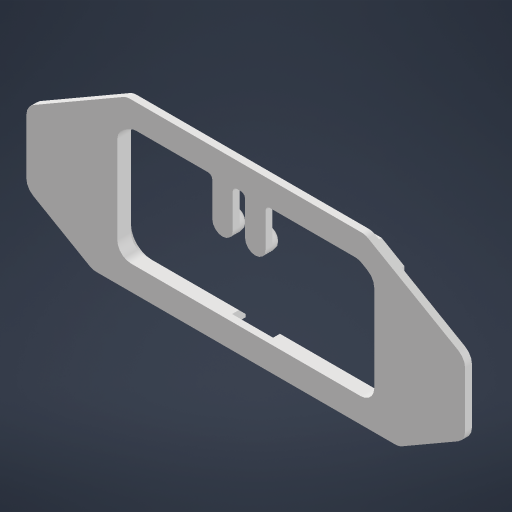
# Autodesk Inventor part: Joystick Top
Saved by Autodesk Inventor 2023.4 (Build 274418000, 418)
## iProperties
Created: 2024-04-17
Part Number: Joystick Top
Material: Generic
Document SubType Name: Modeling
Designer: xSibe
Density: 1 g/cm^3
Appearance: Default
Author: xSibe
Autodesk Inventor part; units mm, degrees
ref_plane "YZ Plane" through (0, 0, 0) normal (1, 0, 0) x (0, 1, 0)
ref_plane "XZ Plane" through (0, 0, 0) normal (0, 1, 0) x (-1, 0, 0)
ref_plane "XY Plane" through (0, 0, 0) normal (0, 0, 1) x (1, 0, 0)
ref_plane "Work Plane1" through (0, 0, 8.5) normal (0, 0, 1) x (1, 0, 0)
sketch "Sketch1" plane through (0, 0, 8.5) normal (0, 0, 1) x (1, 0, 0)
  line L0 (-3.75, -14) -> (-3.75, -11.5) projected
  line L1 (-25.5, -11.5) -> (-3.75, -11.5) projected
  line L2 (-25.5, 11.5) -> (-25.5, -11.5) projected
  line L3 (25.5, -11.5) -> (25.5, 11.5) projected
  line L4 (3.75, -11.5) -> (25.5, -11.5) projected
  line L5 (3.75, -11.5) -> (3.75, -14) projected
  line L6 (27.3301, -14) -> (3.75, -14) projected
  line L7 (-3.75, -14) -> (-27.3301, -14) projected
  line L8 (38.8744, -7.7217) -> (28.5801, -13.6651) projected
  line L9 (-28.5801, -13.6651) -> (-38.8744, -7.7217) projected
  line L10 (40.1244, 10.5622) -> (40.1244, -5.5566) projected
  line L11 (-40.1244, 10.5622) -> (-40.1244, -5.5566) projected
  line L12 (-21.1699, 14) -> (-25.5, 11.5) projected
  line L13 (21.1699, 14) -> (-21.1699, 14) projected
  line L14 (25.5, 11.5) -> (21.1699, 14) projected
  arc A0 (-28.5801, -13.6651) -> (-27.3301, -14) centre (-27.3301, -11.5) ccw projected
  arc A1 (27.3301, -14) -> (28.5801, -13.6651) centre (27.3301, -11.5) ccw projected
  arc A2 (38.8744, -7.7217) -> (40.1244, -5.5566) centre (37.6244, -5.5566) ccw projected
  arc A3 (-40.1244, -5.5566) -> (-38.8744, -7.7217) centre (-37.6244, -5.5566) ccw projected
  line L15 (25.5, -11.5) -> (-25.5, -11.5)
  line L16 (-25.5, -11.5) -> (-25.5, 11.5)
  line L17 (-25.5, 11.5) -> (-21.1699, 14)
  line L18 (-21.1699, 14) -> (21.1699, 14)
  line L19 (21.1699, 14) -> (25.5, 11.5)
  line L20 (25.5, 11.5) -> (25.5, -11.5)
  line L21 (-25.25, -11.25) -> (25.25, -11.25)
  line L22 (25.25, -11.25) -> (25.25, 11.3557)
  line L23 (25.25, 11.3557) -> (21.1029, 13.75)
  line L24 (21.1029, 13.75) -> (-21.1029, 13.75)
  line L25 (-21.1029, 13.75) -> (-25.25, 11.3557)
  line L26 (-25.25, 11.3557) -> (-25.25, -11.25)
  line L27 (-23.5, -9.5) -> (23.5, -9.5)
  line L28 (23.5, -9.5) -> (23.5, 10.3453)
  line L29 (23.5, 10.3453) -> (20.634, 12)
  line L30 (20.634, 12) -> (-20.634, 12)
  line L31 (-20.634, 12) -> (-23.5, 10.3453)
  line L32 (-23.5, 10.3453) -> (-23.5, -9.5)
  line L33 (-28, -14) -> (28, -14)
  line L34 (28, -14) -> (28, 12.9434)
  line L35 (28, 12.9434) -> (21.8397, 16.5)
  line L36 (21.8397, 16.5) -> (-21.8397, 16.5)
  line L37 (-21.8397, 16.5) -> (-28, 12.9434)
  line L38 (-28, 12.9434) -> (-28, -14)
  line L39 (25.25, 0.0528) -> (28, 0.0528)
  line L40 (-25.25, 0.0528) -> (-28, 0.0528)
  line L41 (28, -14) -> (15.8299, -6.9736)
  line L42 (15.8299, -6.9736) -> (15.8299, 7.0792)
  line L43 (15.8299, 7.0792) -> (28, 14.1057)
  line L44 (28, 14.1057) -> (40.1701, 7.0792)
  line L45 (40.1701, 7.0792) -> (40.1701, -6.9736)
  line L46 (40.1701, -6.9736) -> (28, -14)
  line L47 (-28, -14) -> (-40.1701, -6.9736)
  line L48 (-40.1701, -6.9736) -> (-40.1701, 7.0792)
  line L49 (-40.1701, 7.0792) -> (-28, 14.1057)
  line L50 (-28, 14.1057) -> (-15.8299, 7.0792)
  line L51 (-15.8299, 7.0792) -> (-15.8299, -6.9736)
  line L52 (-15.8299, -6.9736) -> (-28, -14)
  line L53 (28, 12.9434) -> (40.1701, 5.917)
  line L54 (-28, 12.9434) -> (-40.1701, 5.917)
  line L55 (3.75, -11.5) -> (-3.75, -11.5)
  line L56 (-3.75, -11.5) -> (-3.75, -9.5)
  line L57 (-3.75, -9.5) -> (3.75, -9.5)
  line L58 (3.75, -9.5) -> (3.75, -11.5)
  arc A4 (36.3744, 8.3971) -> (40.1244, 10.5622) centre (37.6244, 10.5622) ccw projected
  line L59 (36.3744, 8.3971) -> (22.5449, 16.3816) projected
  arc A5 (22.5449, 16.3816) -> (21.1699, 16.75) centre (21.1699, 14) ccw projected
  line L60 (21.1699, 16.75) -> (-21.1699, 16.75) projected
  arc A6 (-21.1699, 16.75) -> (-22.5449, 16.3816) centre (-21.1699, 14) ccw projected
  line L61 (-22.5449, 16.3816) -> (-36.3744, 8.3971) projected
  arc A7 (-40.1244, 10.5622) -> (-36.3744, 8.3971) centre (-37.6244, 10.5622) ccw projected
  point P0 (40.1244, 7)
  point P1 (-40.1244, 7)
  point P2 (3.75, -11.25)
  point P3 (-3.75, -11.25)
  dimension "d15" = 0.25
  dimension "d16" = 2
  dimension "d17" = 2.5
  constraints: 88 end point, 12 perpendicular, 6 point on line, 4 equal length, 2 coincident, 2 collinear, 2 midpoint, 1 horizontal, 41 other
  measures "d15" distance between parallel lines of L15 L21
  measures "d16" distance between parallel lines of L15 L27
  measures "d17" distance between parallel lines of L15 L33
extrude "Extrusion1" add sketch "Sketch1" against normal blind 2.5 contours L21 L52 L27 L56 | L21 L26 L25 L50 L31 L32 L27 L52 | L58 L27 L41 L21 | L41 L27 L28 L29 L43 L23 L22 L21 | L25 L24 L23 L43 L29 L30 L31 L50
sketch "Sketch2" plane through (0, 0, 8.5) normal (0, 0, 1) x (1, 0, 0)
  line L0 (25.25, -11.25) -> (25.25, 11.3557) projected
  line L1 (25.25, 11.3557) -> (21.1029, 13.75) projected
  line L2 (21.1029, 13.75) -> (-21.1029, 13.75) projected
  line L3 (-21.1029, 13.75) -> (-25.25, 11.3557) projected
  line L4 (-25.25, 11.3557) -> (-25.25, -11.25) projected
  line L5 (3.75, -11.25) -> (25.25, -11.25) projected
  line L6 (23.5, -9.5) -> (3.75, -9.5) projected
  line L7 (-23.5, -9.5) -> (-23.5, 10.3453) projected
  line L8 (-23.5, 10.3453) -> (-20.634, 12) projected
  line L9 (-20.634, 12) -> (20.634, 12) projected
  line L10 (20.634, 12) -> (23.5, 10.3453) projected
  line L11 (23.5, 10.3453) -> (23.5, -9.5) projected
  line L12 (3.75, -9.5) -> (3.75, -11.25) projected
  line L13 (-25.25, -11.25) -> (-3.75, -11.25) projected
  line L14 (-3.75, -11.25) -> (-3.75, -9.5) projected
  line L15 (-3.75, -9.5) -> (-23.5, -9.5) projected
  line L16 (25.25, -11.25) -> (-25.25, -11.25)
  line L17 (-25.25, -11.25) -> (-25.25, 11.3557)
  line L18 (-25.25, 11.3557) -> (-21.1029, 13.75)
  line L19 (-21.1029, 13.75) -> (21.1029, 13.75)
  line L20 (21.1029, 13.75) -> (25.25, 11.3557)
  line L21 (25.25, 11.3557) -> (25.25, -11.25)
  line L22 (-23.5, -9.5) -> (23.5, -9.5)
  line L23 (23.5, -9.5) -> (23.5, 10.3453)
  line L24 (23.5, 10.3453) -> (20.634, 12)
  line L25 (20.634, 12) -> (-20.634, 12)
  line L26 (-20.634, 12) -> (-23.5, 10.3453)
  line L27 (-23.5, 10.3453) -> (-23.5, -9.5)
  line L28 (-25.5, -11.5) -> (25.5, -11.5)
  line L29 (25.5, -11.5) -> (25.5, 11.5)
  line L30 (25.5, 11.5) -> (21.1699, 14)
  line L31 (21.1699, 14) -> (-21.1699, 14)
  line L32 (-21.1699, 14) -> (-25.5, 11.5)
  line L33 (-25.5, 11.5) -> (-25.5, -11.5)
  line L34 (28, -14) -> (-28, -14)
  line L35 (-28, -14) -> (-28, 12.9434)
  line L36 (-28, 12.9434) -> (-21.8397, 16.5)
  line L37 (-21.8397, 16.5) -> (21.8397, 16.5)
  line L38 (21.8397, 16.5) -> (28, 12.9434)
  line L39 (28, 12.9434) -> (28, -14)
  line L40 (28, -14) -> (28, 0)
  line L41 (-28, -14) -> (-28, 0)
  line L42 (28, -14) -> (15.8756, -7)
  line L43 (15.8756, -7) -> (15.8756, 7)
  line L44 (15.8756, 7) -> (28, 14)
  line L45 (28, 14) -> (40.1244, 7)
  line L46 (40.1244, 7) -> (40.1244, -7)
  line L47 (40.1244, -7) -> (28, -14)
  line L48 (-28, -14) -> (-40.1244, -7)
  line L49 (-40.1244, -7) -> (-40.1244, 7)
  line L50 (-40.1244, 7) -> (-28, 14)
  line L51 (-28, 14) -> (-15.8756, 7)
  line L52 (-15.8756, 7) -> (-15.8756, -7)
  line L53 (-15.8756, -7) -> (-28, -14)
  line L54 (28, 12.9434) -> (40.1244, 5.9434)
  line L55 (-28, 12.9434) -> (-40.1244, 5.9434)
  line L56 (-1.25, 5) -> (1.75, 5)
  line L57 (1.75, 5) -> (-4.25, 5)
  circle A0 centre (1.75, 5) radius 1.875
  circle A1 centre (-4.25, 5) radius 1.875
  line L58 (1.75, 5) -> (1.75, 12) construction
  line L59 (3.625, 5) -> (3.625, 12)
  line L60 (-0.125, 12) -> (-0.125, 5)
  arc A2 (-0.125, 5) -> (3.625, 5) centre (1.75, 5) ccw
  arc A3 (3.625, 12) -> (-0.125, 12) centre (1.75, 12) ccw
  line L61 (-4.25, 5) -> (-4.25, 12) construction
  line L62 (-6.125, 5) -> (-6.125, 12)
  line L63 (-2.375, 12) -> (-2.375, 5)
  arc A4 (-6.125, 5) -> (-2.375, 5) centre (-4.25, 5) ccw
  arc A5 (-2.375, 12) -> (-6.125, 12) centre (-4.25, 12) ccw
  line L64 (0, 12) -> (0, 5)
  line L65 (0, 5) -> (-1.25, 5)
  point P0 (1.75, 8.5)
  point P1 (-4.25, 8.5)
  point P2 (-0.125, 12)
  point P3 (-0.125, 5)
  point P4 (3.625, 5)
  point P5 (3.625, 12)
  point P6 (-2.375, 5)
  point P7 (-2.375, 12)
  point P8 (-6.125, 12)
  point P9 (-6.125, 5)
  dimension "d18" = 1.75
  dimension "d19" = 0.25
  dimension "d20" = 2.5
  dimension "d21" = 14
  dimension "d22" = 14
  dimension "d30" = 3
  dimension "d31" = 6
  dimension "d32" = 3.75
  dimension "d33" = 3.75
  dimension "d37" = 7
  dimension "d38" = 1.25
  constraints: 104 end point, 11 perpendicular, 10 tangent, 8 point on circle, 7 point on line, 6 centre point, 6 collinear, 4 coincident, 3 midpoint, 2 parallel, 1 horizontal, 1 vertical, 41 other
  measures "d18" distance between parallel lines of L16 L22
  measures "d19" distance between parallel lines of L16 L28
  measures "d20" distance between parallel lines of L28 L34
  measures "d21" distance of L34.start L40.end
  measures "d22" distance of L34.end L41.end
  measures "d30" distance of L56.start L56.end
  measures "d31" distance of L56.end L57.end
  measures "d32" diameter of A0
  measures "d33" diameter of A1
  measures "d37" distance of L64.start L64.end
  measures "d38" distance of L64.end L56.start
extrude "Extrusion2" add sketch "Sketch2" along normal blind 1.25 contours L5 L42 L6 L11 L10 L44 L1 L0 | L0 L1 L44 L30 L29 L28 L42 L5 | L42 L28 L53 L13 L16 L5 | L5 L12 L6 L42 | L44 L10 L9 A3 L2 L1 | L1 L2 A3 A5 L3 L51 L32 L31 L30 L44 | L16 L14 L22 L12 | L42 L34 L53 L28 | L28 L29 L30 L44 L38 L39 L42 | L30 L31 L32 L51 L36 L37 L38 L44 | L13 L53 L15 L14 | L53 L35 L36 L51 L32 L33 L28 | L28 L33 L32 L51 L3 L4 L13 L53 | L39 L54 L46 L47 | A3 L9 L2 | L2 A3 | L13 L4 L3 L51 L8 L7 L15 L53 | L48 L49 L55 L35 | A3 L9 A5 L2 | L59 A0 L64 L9 | A5 L9 L2 | L2 A5 | L9 L64 A0 L60 | A0 L56 L64 | A5 L9 L8 L51 L3 L2 | L63 A1 L62 L9 | A0 L64 L56 | A1
extrude "Extrusion3" add sketch "Sketch2" against normal blind 1.5 contours A0 L56 L64 | A0 L64 L56 | A1
fillet "Fillet1" radius 2.5 14 edges at (40.1244, -7, 9.125) (40.1244, 5.9434, 9.125) (28, -14, 9.125) (-28, -14, 9.125) (-40.1244, -7, 9.125) (-40.1244, 5.9434, 9.125) (-21.8397, 16.5, 9.125) (21.8397, 16.5, 9.125) (23.5, -9.5, 7.875) (23.5, 10.3453, 7.875) (20.634, 12, 7.875) (-23.5, -9.5, 7.875) (-23.5, 10.3453, 7.875) (-20.634, 12, 7.875)
chamfer "Chamfer1" distance 1.25 angle 45 13 edges at (-12.375, -9.5, 6) (-22.7678, -8.7678, 6) (-23.5, 0.951, 6) (-23.1651, 10.1519, 6) (-21.7321, 11.366, 6) (-20.6111, 11.9148, 6) (0, 12, 6) (20.6111, 11.9148, 6) (21.7321, 11.366, 6) (23.1651, 10.1519, 6) (23.5, 0.951, 6) (22.7678, -8.7678, 6) (12.375, -9.5, 6)
fillet "Fillet2" radius 0.75 8 edges at (-6.125, 12, 9.125) (-0.125, 12, 9.125) (-2.375, 12, 9.125) (3.625, 12, 9.125) (-0.125, 5, 7) (-6.125, 5, 7) (-4.25, 12, 8.5) (1.75, 12, 8.5)
body "Solid1"
